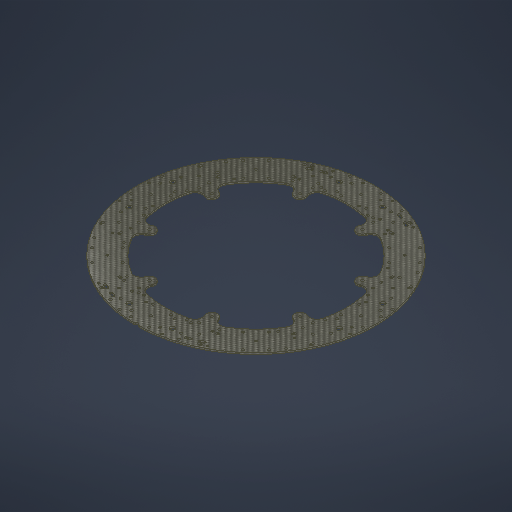
# Autodesk Inventor part: Body_Outer_Plate
Saved by Autodesk Inventor 2025 (Build 290162010, 162A)
## iProperties
Created: 2023-12-04
Part Number: Body_Outer_Plate
Material: CFRP
Document SubType Name: Modeling
Designer: dzw04
Density: 1.43 g/cm^3
Appearance: Carbon Fiber 1
Mass: 106.561 g
Surface Area: 824.877 cm^2
Volume: 74.5179 cm^3
Author: dzw04
Autodesk Inventor part; units mm, degrees
ref_plane "YZ Plane" through (0, 0, 0) normal (1, 0, 0) x (0, 1, 0)
ref_plane "XZ Plane" through (0, 0, 0) normal (0, 1, 0) x (-1, 0, 0)
ref_plane "XY Plane" through (0, 0, 0) normal (0, 0, 1) x (1, 0, 0)
sketch "Sketch1" plane through (0, 0, 0) normal (0, 1, 0) x (-1, 0, 0)
  arc A0 (286.4193, 194.7045) -> (272.8789, 201.567) centre (276.7057, 192.3282) ccw
  arc A1 (201.1228, 271.8066) -> (214.981, 266.0663) centre (208.0519, 268.9364) ccw
  line L0 (215.4252, 267.1386) -> (214.981, 266.0663)
  arc A2 (229.8521, 271.8607) -> (215.4252, 267.1386) centre (224.664, 263.3118) ccw
  circle A3 centre (39.4263, 92.5) radius 1.6
  circle A4 centre (61.0636, 208.0519) radius 1.6
  circle A5 centre (165, 310) radius 1.6
  arc A6 (271.8607, 229.8521) -> (229.8521, 271.8607) centre (165, 165) ccw
  circle A7 centre (267.5305, 62.4695) radius 1.6
  arc A8 (58.1393, 229.8521) -> (62.8614, 215.4252) centre (66.6882, 224.664) ccw
  arc A9 (267.1386, 215.4252) -> (271.8607, 229.8521) centre (263.3118, 224.664) ccw
  line L1 (266.0663, 214.981) -> (267.1386, 215.4252)
  circle A10 centre (290.5737, 92.5) radius 1.6
  arc A11 (266.0663, 214.981) -> (271.8066, 201.1228) centre (268.9364, 208.0519) ccw
  line L2 (272.8789, 201.567) -> (271.8066, 201.1228)
  circle A12 centre (109.5109, 298.9625) radius 1.6
  line L3 (201.567, 57.1211) -> (201.1228, 58.1934)
  circle A13 centre (121.9481, 268.9364) radius 1.6
  arc A14 (286.4193, 135.2955) -> (286.4193, 194.7045) centre (165, 165) ccw
  arc A15 (272.8789, 128.433) -> (286.4193, 135.2955) centre (276.7057, 137.6718) ccw
  circle A16 centre (31.0375, 109.5109) radius 1.6
  line L4 (271.8066, 128.8772) -> (272.8789, 128.433)
  arc A17 (271.8066, 128.8772) -> (266.0663, 115.019) centre (268.9364, 121.9481) ccw
  circle A18 centre (109.5109, 31.0375) radius 1.6
  circle A19 centre (62.4695, 267.5305) radius 1.6
  line L5 (267.1386, 114.5748) -> (266.0663, 115.019)
  arc A20 (271.8607, 100.1479) -> (267.1386, 114.5748) centre (263.3118, 105.336) ccw
  arc A21 (229.8521, 58.1393) -> (271.8607, 100.1479) centre (165, 165) ccw
  circle A22 centre (268.9364, 208.0519) radius 1.6
  arc A23 (215.4252, 62.8614) -> (229.8521, 58.1393) centre (224.664, 66.6882) ccw
  line L6 (214.981, 63.9337) -> (215.4252, 62.8614)
  arc A24 (214.981, 63.9337) -> (201.1228, 58.1934) centre (208.0519, 61.0636) ccw
  line L7 (62.8614, 215.4252) -> (63.9337, 214.981)
  arc A25 (194.7045, 43.5807) -> (201.567, 57.1211) centre (192.3282, 53.2943) ccw
  arc A26 (135.2955, 43.5807) -> (194.7045, 43.5807) centre (165, 165) ccw
  arc A27 (128.433, 57.1211) -> (135.2955, 43.5807) centre (137.6718, 53.2943) ccw
  line L8 (128.8772, 58.1934) -> (128.433, 57.1211)
  circle A28 centre (39.4263, 237.5) radius 1.6
  circle A29 centre (31.0375, 220.4891) radius 1.6
  arc A30 (58.1934, 201.1228) -> (63.9337, 214.981) centre (61.0636, 208.0519) ccw
  arc A31 (128.8772, 58.1934) -> (115.019, 63.9337) centre (121.9481, 61.0636) ccw
  circle A32 centre (62.4695, 62.4695) radius 1.6
  line L9 (114.5748, 62.8614) -> (115.019, 63.9337)
  circle A33 centre (20, 165) radius 1.6
  arc A34 (100.1479, 58.1393) -> (114.5748, 62.8614) centre (105.336, 66.6882) ccw
  circle A35 centre (267.5305, 267.5305) radius 1.6
  line L10 (58.1934, 201.1228) -> (57.1211, 201.567)
  arc A36 (57.1211, 201.567) -> (43.5807, 194.7045) centre (53.2943, 192.3282) ccw
  circle A37 centre (61.0636, 121.9481) radius 1.6
  circle A38 centre (298.9625, 220.4891) radius 1.6
  arc A39 (43.5807, 194.7045) -> (43.5807, 135.2955) centre (165, 165) ccw
  arc A40 (43.5807, 135.2955) -> (57.1211, 128.433) centre (53.2943, 137.6718) ccw
  line L11 (57.1211, 128.433) -> (58.1934, 128.8772)
  arc A41 (63.9337, 115.019) -> (58.1934, 128.8772) centre (61.0636, 121.9481) ccw
  circle A42 centre (208.0519, 61.0636) radius 1.6
  circle A43 centre (298.9625, 109.5109) radius 1.6
  circle A44 centre (220.4891, 31.0375) radius 1.6
  line L12 (63.9337, 115.019) -> (62.8614, 114.5748)
  circle A45 centre (165, 20) radius 1.6
  arc A46 (62.8614, 114.5748) -> (58.1393, 100.1479) centre (66.6882, 105.336) ccw
  circle A47 centre (208.0519, 268.9364) radius 1.6
  arc A48 (58.1393, 100.1479) -> (100.1479, 58.1393) centre (165, 165) ccw
  circle A49 centre (268.9364, 121.9481) radius 1.6
  circle A50 centre (310, 165) radius 1.6
  arc A51 (162.8516, 328.7216) -> (167.1484, 328.7216) centre (165, 330) ccw
  arc A52 (162.8516, 328.7216) -> (160.6371, 329.9423) centre (160.7032, 327.4432) ccw
  arc A53 (169.3629, 329.9423) -> (167.1484, 328.7216) centre (169.2968, 327.4432) ccw
  line L13 (115.019, 266.0663) -> (114.5748, 267.1386)
  circle A54 centre (290.5737, 237.5) radius 1.6
  circle A55 centre (220.4891, 298.9625) radius 1.6
  circle A56 centre (121.9481, 61.0636) radius 1.6
  arc A57 (160.6371, 329.9423) -> (169.3629, 329.9423) centre (165, 165) ccw
  circle A58 centre (135.5551, 323.917) radius 1.6
  circle A59 centre (135.5551, 289.917) radius 1.6
  circle A60 centre (194.4449, 289.917) radius 1.6
  circle A61 centre (194.4449, 323.917) radius 1.6
  circle A62 centre (6.083, 135.5551) radius 1.6
  circle A63 centre (40.083, 135.5551) radius 1.6
  circle A64 centre (40.083, 194.4449) radius 1.6
  circle A65 centre (6.083, 194.4449) radius 1.6
  circle A66 centre (194.4449, 6.083) radius 1.6
  circle A67 centre (194.4449, 40.083) radius 1.6
  circle A68 centre (135.5551, 40.083) radius 1.6
  circle A69 centre (135.5551, 6.083) radius 1.6
  circle A70 centre (323.917, 194.4449) radius 1.6
  circle A71 centre (289.917, 194.4449) radius 1.6
  circle A72 centre (289.917, 135.5551) radius 1.6
  circle A73 centre (323.917, 135.5551) radius 1.6
  arc A74 (201.567, 272.8789) -> (194.7045, 286.4193) centre (192.3282, 276.7057) ccw
  line L14 (201.1228, 271.8066) -> (201.567, 272.8789)
  arc A75 (194.7045, 286.4193) -> (135.2955, 286.4193) centre (165, 165) ccw
  arc A76 (135.2955, 286.4193) -> (128.433, 272.8789) centre (137.6718, 276.7057) ccw
  line L15 (128.433, 272.8789) -> (128.8772, 271.8066)
  arc A77 (115.019, 266.0663) -> (128.8772, 271.8066) centre (121.9481, 268.9364) ccw
  arc A78 (114.5748, 267.1386) -> (100.1479, 271.8607) centre (105.336, 263.3118) ccw
  arc A79 (100.1479, 271.8607) -> (58.1393, 229.8521) centre (165, 165) ccw
  circle A80 centre (212.3712, 318.561) radius 1.6
  circle A81 centre (200.8907, 39.1554) radius 1.6
  circle A82 centre (117.6288, 318.561) radius 1.6
  circle A83 centre (89.9125, 307.0805) radius 1.6
  circle A84 centre (101.393, 279.3641) radius 1.6
  circle A85 centre (200.8907, 290.8446) radius 1.6
  circle A86 centre (104.0989, 285.8969) radius 1.6
  circle A87 centre (129.1093, 290.8446) radius 1.6
  circle A88 centre (240.0875, 307.0805) radius 1.6
  circle A89 centre (228.607, 279.3641) radius 1.6
  circle A90 centre (225.9011, 285.8969) radius 1.6
  circle A91 centre (207.4235, 293.5506) radius 1.6
  circle A92 centre (117.6288, 11.439) radius 1.6
  circle A93 centre (89.9125, 22.9195) radius 1.6
  circle A94 centre (101.393, 50.6359) radius 1.6
  circle A95 centre (104.0989, 44.1031) radius 1.6
  circle A96 centre (122.5765, 36.4494) radius 1.6
  circle A97 centre (129.1093, 39.1554) radius 1.6
  circle A98 centre (212.3712, 11.439) radius 1.6
  circle A99 centre (240.0875, 22.9195) radius 1.6
  circle A100 centre (228.607, 50.6359) radius 1.6
  circle A101 centre (225.9011, 44.1031) radius 1.6
  circle A102 centre (207.4235, 36.4494) radius 1.6
  line L16 (17.2755, 136.1225) -> (17.2755, 133.8775)
  line L17 (17.2755, 196.1225) -> (17.2755, 193.8775)
  arc A103 (18.3955, 192.0815) -> (18.3955, 197.9185) centre (19.8255, 195) ccw
  arc A104 (132.0815, 311.6045) -> (137.9185, 311.6045) centre (135, 310.1745) ccw
  arc A105 (192.0815, 311.6045) -> (197.9185, 311.6045) centre (195, 310.1745) ccw
  line L18 (196.1225, 312.7245) -> (193.8775, 312.7245)
  arc A106 (311.6045, 197.9185) -> (311.6045, 192.0815) centre (310.1745, 195) ccw
  line L19 (312.7245, 193.8775) -> (312.7245, 196.1225)
  arc A107 (311.6045, 137.9185) -> (311.6045, 132.0815) centre (310.1745, 135) ccw
  line L20 (312.7245, 133.8775) -> (312.7245, 136.1225)
  arc A108 (197.9185, 18.3955) -> (192.0815, 18.3955) centre (195, 19.8255) ccw
  line L21 (193.8775, 17.2755) -> (196.1225, 17.2755)
  line L22 (133.8775, 17.2755) -> (136.1225, 17.2755)
  arc A109 (137.9185, 18.3955) -> (132.0815, 18.3955) centre (135, 19.8255) ccw
  line L23 (136.1225, 312.7245) -> (133.8775, 312.7245)
  arc A110 (18.3955, 132.0815) -> (18.3955, 137.9185) centre (19.8255, 135) ccw
  circle A111 centre (32.6859, 255.8253) radius 1.6
  circle A112 centre (152.5, 295) radius 1.6
  circle A113 centre (64.2373, 81.915) radius 1.6
  circle A114 centre (60.7017, 286.9759) radius 1.6
  circle A115 centre (43.0241, 269.2983) radius 1.6
  circle A116 centre (58.6667, 89.1747) radius 1.6
  circle A117 centre (297.3141, 74.1747) radius 1.6
  circle A118 centre (81.915, 64.2373) radius 1.6
  circle A119 centre (269.2983, 286.9759) radius 1.6
  circle A120 centre (43.0241, 60.7017) radius 1.6
  circle A121 centre (152.5, 35) radius 1.6
  circle A122 centre (81.915, 265.7627) radius 1.6
  circle A123 centre (295, 152.5) radius 1.6
  circle A124 centre (177.5, 35) radius 1.6
  circle A125 centre (283.8333, 219.1747) radius 1.6
  circle A126 centre (64.2373, 248.085) radius 1.6
  circle A127 centre (271.3333, 240.8253) radius 1.6
  circle A128 centre (297.3141, 255.8253) radius 1.6
  circle A129 centre (5, 152.5) radius 1.6
  circle A130 centre (283.8333, 110.8253) radius 1.6
  circle A131 centre (295, 177.5) radius 1.6
  circle A132 centre (177.5, 5) radius 1.6
  circle A133 centre (271.3333, 89.1747) radius 1.6
  circle A134 centre (286.9759, 269.2983) radius 1.6
  circle A135 centre (177.5, 295) radius 1.6
  circle A136 centre (60.7017, 43.0241) radius 1.6
  circle A137 centre (325, 152.5) radius 1.6
  circle A138 centre (152.5, 325) radius 1.6
  circle A139 centre (325, 177.5) radius 1.6
  circle A140 centre (32.6859, 74.1747) radius 1.6
  circle A141 centre (35, 152.5) radius 1.6
  circle A142 centre (286.9759, 60.7017) radius 1.6
  circle A143 centre (265.7627, 81.915) radius 1.6
  circle A144 centre (46.1667, 110.8253) radius 1.6
  circle A145 centre (269.2983, 43.0241) radius 1.6
  circle A146 centre (265.7627, 248.085) radius 1.6
  circle A147 centre (152.5, 5) radius 1.6
  circle A148 centre (248.085, 64.2373) radius 1.6
  circle A149 centre (177.5, 325) radius 1.6
  circle A150 centre (46.1667, 219.1747) radius 1.6
  circle A151 centre (35, 177.5) radius 1.6
  circle A152 centre (5, 177.5) radius 1.6
  circle A153 centre (58.6667, 240.8253) radius 1.6
  circle A154 centre (248.085, 265.7627) radius 1.6
  arc A155 (308.4, 231.6) -> (311.6, 231.6) centre (310, 231.6) ccw
  arc A156 (311.6, 233.4) -> (311.4139, 234.149) centre (310, 233.4) ccw
  line L24 (311.6, 233.4) -> (311.6, 231.6)
  arc A157 (18.5861, 95.851) -> (21.5998, 96.5743) centre (20.1859, 95.8253) ccw
  line L25 (308.4, 231.6) -> (308.4, 233.4)
  arc A158 (308.4002, 233.4257) -> (308.4, 233.4) centre (310, 233.4) ccw
  arc A159 (311.4139, 234.149) -> (308.4002, 233.4257) centre (309.8141, 234.1747) ccw
  arc A160 (311.4139, 95.851) -> (311.6, 96.6) centre (310, 96.6) ccw
  line L26 (311.6, 96.6) -> (311.6, 98.4)
  arc A161 (311.6, 98.4) -> (308.4, 98.4) centre (310, 98.4) ccw
  line L27 (308.4, 98.4) -> (308.4, 96.6)
  arc A162 (308.4, 96.6) -> (308.4002, 96.5743) centre (310, 96.6) ccw
  arc A163 (308.4002, 96.5743) -> (311.4139, 95.851) centre (309.8141, 95.8253) ccw
  arc A164 (18.5861, 234.149) -> (18.4, 233.4) centre (20, 233.4) ccw
  line L28 (18.4, 233.4) -> (18.4, 231.6)
  arc A165 (18.4, 231.6) -> (21.6, 231.6) centre (20, 231.6) ccw
  line L29 (21.6, 231.6) -> (21.6, 233.4)
  arc A166 (21.6, 233.4) -> (21.5998, 233.4257) centre (20, 233.4) ccw
  arc A167 (21.5998, 233.4257) -> (18.5861, 234.149) centre (20.1859, 234.1747) ccw
  arc A168 (18.4, 96.6) -> (18.5861, 95.851) centre (20, 96.6) ccw
  line L30 (18.4, 96.6) -> (18.4, 98.4)
  arc A169 (21.6, 98.4) -> (18.4, 98.4) centre (20, 98.4) ccw
  line L31 (21.6, 98.4) -> (21.6, 96.6)
  arc A170 (21.5998, 96.5743) -> (21.6, 96.6) centre (20, 96.6) ccw
  arc A171 (231.6, 311.6) -> (231.6, 308.4) centre (231.6, 310) ccw
  arc A172 (98.4, 308.4) -> (98.4, 311.6) centre (98.4, 310) ccw
  line L32 (98.4, 311.6) -> (96.6, 311.6)
  arc A173 (96.6, 21.6) -> (96.6, 18.4) centre (96.6, 20) ccw
  circle A174 centre (123.4, 20) radius 1.6
  arc A175 (96.6, 286.6) -> (96.6, 283.4) centre (96.6, 285) ccw
  line L33 (96.6, 283.4) -> (98.4, 283.4)
  arc A176 (98.4, 283.4) -> (98.4, 286.6) centre (98.4, 285) ccw
  line L34 (98.4, 286.6) -> (96.6, 286.6)
  circle A177 centre (310, 206.6) radius 1.6
  circle A178 centre (285, 206.6) radius 1.6
  arc A179 (283.4, 231.6) -> (286.6, 231.6) centre (285, 231.6) ccw
  line L35 (286.6, 231.6) -> (286.6, 233.4)
  arc A180 (286.6, 233.4) -> (283.4, 233.4) centre (285, 233.4) ccw
  arc A181 (233.4, 43.4) -> (233.4, 46.6) centre (233.4, 45) ccw
  line L36 (283.4, 233.4) -> (283.4, 231.6)
  circle A182 centre (206.6, 45) radius 1.6
  circle A183 centre (206.6, 20) radius 1.6
  arc A184 (233.4, 18.4) -> (233.4, 21.6) centre (233.4, 20) ccw
  line L37 (233.4, 21.6) -> (231.6, 21.6)
  arc A185 (231.6, 21.6) -> (231.6, 18.4) centre (231.6, 20) ccw
  circle A186 centre (123.4, 45) radius 1.6
  line L38 (231.6, 43.4) -> (233.4, 43.4)
  arc A187 (231.6, 46.6) -> (231.6, 43.4) centre (231.6, 45) ccw
  circle A188 centre (206.6, 285) radius 1.6
  circle A189 centre (206.6, 310) radius 1.6
  arc A190 (233.4, 308.4) -> (233.4, 311.6) centre (233.4, 310) ccw
  line L39 (233.4, 308.4) -> (231.6, 308.4)
  line L40 (231.6, 18.4) -> (233.4, 18.4)
  line L41 (231.6, 311.6) -> (233.4, 311.6)
  arc A191 (233.4, 283.4) -> (233.4, 286.6) centre (233.4, 285) ccw
  line L42 (233.4, 283.4) -> (231.6, 283.4)
  arc A192 (231.6, 286.6) -> (231.6, 283.4) centre (231.6, 285) ccw
  line L43 (233.4, 46.6) -> (231.6, 46.6)
  circle A193 centre (123.4, 285) radius 1.6
  circle A194 centre (123.4, 310) radius 1.6
  arc A195 (96.6, 311.6) -> (96.6, 308.4) centre (96.6, 310) ccw
  line L44 (96.6, 308.4) -> (98.4, 308.4)
  line L45 (96.6, 21.6) -> (98.4, 21.6)
  arc A196 (98.4, 18.4) -> (98.4, 21.6) centre (98.4, 20) ccw
  line L46 (98.4, 18.4) -> (96.6, 18.4)
  arc A197 (96.6, 46.6) -> (96.6, 43.4) centre (96.6, 45) ccw
  line L47 (96.6, 46.6) -> (98.4, 46.6)
  arc A198 (98.4, 43.4) -> (98.4, 46.6) centre (98.4, 45) ccw
  line L48 (98.4, 43.4) -> (96.6, 43.4)
  circle A199 centre (310, 123.4) radius 1.6
  circle A200 centre (285, 123.4) radius 1.6
  arc A201 (286.6, 98.4) -> (283.4, 98.4) centre (285, 98.4) ccw
  line L49 (286.6, 98.4) -> (286.6, 96.6)
  arc A202 (283.4, 96.6) -> (286.6, 96.6) centre (285, 96.6) ccw
  line L50 (283.4, 96.6) -> (283.4, 98.4)
  line L51 (231.6, 286.6) -> (233.4, 286.6)
  circle A203 centre (20, 206.6) radius 1.6
  circle A204 centre (45, 206.6) radius 1.6
  arc A205 (43.4, 231.6) -> (46.6, 231.6) centre (45, 231.6) ccw
  line L52 (43.4, 231.6) -> (43.4, 233.4)
  arc A206 (46.6, 233.4) -> (43.4, 233.4) centre (45, 233.4) ccw
  line L53 (46.6, 233.4) -> (46.6, 231.6)
  circle A207 centre (20, 123.4) radius 1.6
  circle A208 centre (45, 123.4) radius 1.6
  arc A209 (46.6, 98.4) -> (43.4, 98.4) centre (45, 98.4) ccw
  line L54 (43.4, 98.4) -> (43.4, 96.6)
  arc A210 (43.4, 96.6) -> (46.6, 96.6) centre (45, 96.6) ccw
  line L55 (46.6, 96.6) -> (46.6, 98.4)
  arc A211 (97.0576, 27.1037) -> (95.833, 24.1473) centre (96.4453, 25.6255) ccw
  line L56 (97.0576, 27.1037) -> (101.677, 25.1903)
  arc A212 (100.4524, 22.2339) -> (101.677, 25.1903) centre (101.0647, 23.7121) ccw
  arc A213 (214.4648, 19.45) -> (215.6894, 16.4936) centre (215.0771, 17.9718) ccw
  arc A214 (220.3088, 18.407) -> (219.0842, 21.3635) centre (219.6965, 19.8853) ccw
  line L57 (220.3088, 18.407) -> (215.6894, 16.4936)
  arc A215 (228.323, 25.1903) -> (229.5476, 22.2339) centre (228.9353, 23.7121) ccw
  arc A216 (115.5352, 310.55) -> (114.3106, 313.5064) centre (114.9229, 312.0282) ccw
  line L58 (110.9158, 308.6365) -> (115.5352, 310.55)
  arc A217 (109.6912, 311.593) -> (110.9158, 308.6365) centre (110.3035, 310.1147) ccw
  line L59 (228.323, 25.1903) -> (232.9424, 27.1037)
  arc A218 (234.167, 24.1473) -> (232.9424, 27.1037) centre (233.5547, 25.6255) ccw
  line L60 (234.167, 24.1473) -> (229.5476, 22.2339)
  line L61 (214.4648, 19.45) -> (219.0842, 21.3635)
  arc A219 (232.9424, 302.8963) -> (234.167, 305.8527) centre (233.5547, 304.3745) ccw
  line L62 (228.323, 304.8097) -> (232.9424, 302.8963)
  line L63 (114.3106, 313.5064) -> (109.6912, 311.593)
  arc A220 (101.677, 304.8097) -> (100.4524, 307.7661) centre (101.0647, 306.2879) ccw
  line L64 (97.0576, 302.8963) -> (101.677, 304.8097)
  arc A221 (95.833, 305.8527) -> (97.0576, 302.8963) centre (96.4453, 304.3745) ccw
  line L65 (100.4524, 307.7661) -> (95.833, 305.8527)
  arc A222 (229.5476, 307.7661) -> (228.323, 304.8097) centre (228.9353, 306.2879) ccw
  line L66 (114.3106, 16.4936) -> (109.6912, 18.407)
  arc A223 (110.9158, 21.3635) -> (109.6912, 18.407) centre (110.3035, 19.8853) ccw
  line L67 (110.9158, 21.3635) -> (115.5352, 19.45)
  arc A224 (114.3106, 16.4936) -> (115.5352, 19.45) centre (114.9229, 17.9718) ccw
  line L68 (100.4524, 22.2339) -> (95.833, 24.1473)
  line L69 (220.3088, 311.593) -> (215.6894, 313.5064)
  arc A225 (219.0842, 308.6365) -> (220.3088, 311.593) centre (219.6965, 310.1147) ccw
  line L70 (214.4648, 310.55) -> (219.0842, 308.6365)
  arc A226 (215.6894, 313.5064) -> (214.4648, 310.55) centre (215.0771, 312.0282) ccw
  line L71 (234.167, 305.8527) -> (229.5476, 307.7661)
  circle A227 centre (185, 296.917) radius 1.6
  circle A228 centre (185, 33.083) radius 1.6
  circle A229 centre (33.083, 185) radius 1.6
  circle A230 centre (145, 316.917) radius 1.6
  circle A231 centre (185, 13.083) radius 1.6
  circle A232 centre (13.083, 185) radius 1.6
  circle A233 centre (33.083, 145) radius 1.6
  circle A234 centre (13.083, 145) radius 1.6
  circle A235 centre (185, 316.917) radius 1.6
  circle A236 centre (145, 13.083) radius 1.6
  circle A237 centre (316.917, 185) radius 1.6
  circle A238 centre (296.917, 185) radius 1.6
  circle A239 centre (296.917, 145) radius 1.6
  circle A240 centre (316.917, 145) radius 1.6
  circle A241 centre (145, 33.083) radius 1.6
  circle A242 centre (145, 296.917) radius 1.6
  arc A243 (311.6045, 132.0815) -> (312.7245, 133.8775) centre (310.7245, 133.8775) ccw
  arc A244 (312.7245, 136.1225) -> (311.6045, 137.9185) centre (310.7245, 136.1225) ccw
  arc A245 (312.7245, 196.1225) -> (311.6045, 197.9185) centre (310.7245, 196.1225) ccw
  arc A246 (311.6045, 192.0815) -> (312.7245, 193.8775) centre (310.7245, 193.8775) ccw
  arc A247 (197.9185, 311.6045) -> (196.1225, 312.7245) centre (196.1225, 310.7245) ccw
  arc A248 (193.8775, 312.7245) -> (192.0815, 311.6045) centre (193.8775, 310.7245) ccw
  arc A249 (137.9185, 311.6045) -> (136.1225, 312.7245) centre (136.1225, 310.7245) ccw
  arc A250 (133.8775, 312.7245) -> (132.0815, 311.6045) centre (133.8775, 310.7245) ccw
  arc A251 (18.3955, 197.9185) -> (17.2755, 196.1225) centre (19.2755, 196.1225) ccw
  arc A252 (17.2755, 193.8775) -> (18.3955, 192.0815) centre (19.2755, 193.8775) ccw
  arc A253 (17.2755, 133.8775) -> (18.3955, 132.0815) centre (19.2755, 133.8775) ccw
  arc A254 (18.3955, 137.9185) -> (17.2755, 136.1225) centre (19.2755, 136.1225) ccw
  arc A255 (132.0815, 18.3955) -> (133.8775, 17.2755) centre (133.8775, 19.2755) ccw
  arc A256 (136.1225, 17.2755) -> (137.9185, 18.3955) centre (136.1225, 19.2755) ccw
  arc A257 (192.0815, 18.3955) -> (193.8775, 17.2755) centre (193.8775, 19.2755) ccw
  arc A258 (196.1225, 17.2755) -> (197.9185, 18.3955) centre (196.1225, 19.2755) ccw
  point P0 (17.2755, 137.0149)
  point P1 (17.2755, 132.9851)
  point P2 (17.2755, 197.0149)
  point P3 (17.2755, 192.9851)
  point P4 (17.2755, 192.9851)
  point P5 (17.2755, 197.0149)
  point P6 (132.9851, 312.7245)
  point P7 (137.0149, 312.7245)
  point P8 (192.9851, 312.7245)
  point P9 (197.0149, 312.7245)
  point P10 (197.0149, 312.7245)
  point P11 (192.9851, 312.7245)
  point P12 (312.7245, 197.0149)
  point P13 (312.7245, 192.9851)
  point P14 (312.7245, 192.9851)
  point P15 (312.7245, 197.0149)
  point P16 (312.7245, 137.0149)
  point P17 (312.7245, 132.9851)
  point P18 (312.7245, 132.9851)
  point P19 (312.7245, 137.0149)
  point P20 (197.0149, 17.2755)
  point P21 (192.9851, 17.2755)
  point P22 (192.9851, 17.2755)
  point P23 (197.0149, 17.2755)
  point P24 (132.9851, 17.2755)
  point P25 (137.0149, 17.2755)
  point P26 (137.0149, 17.2755)
  point P27 (132.9851, 17.2755)
  point P28 (137.0149, 312.7245)
  point P29 (132.9851, 312.7245)
  point P30 (17.2755, 132.9851)
  point P31 (17.2755, 137.0149)
  point P32 (167.1484, 328.7216)
  point P33 (100.4524, 307.7661)
  point P34 (232.9424, 302.8963)
  point P35 (234.167, 305.8527)
  point P36 (109.6912, 311.593)
  point P37 (114.3106, 313.5064)
  point P38 (234.167, 24.1473)
  point P39 (229.5476, 22.2339)
  point P40 (215.6894, 16.4936)
  point P41 (214.4648, 19.45)
  point P42 (219.0842, 21.3635)
  point P43 (95.833, 24.1473)
  point P44 (97.0576, 27.1037)
  point P45 (46.6, 98.4)
  point P46 (46.6, 96.6)
  point P47 (46.6, 233.4)
  point P48 (46.6, 231.6)
  point P49 (18.5861, 234.149)
  point P50 (308.4002, 96.5743)
  point P51 (21.5998, 96.5743)
  point P52 (137.0149, 17.2755)
  point P53 (132.9851, 17.2755)
  point P54 (192.9851, 17.2755)
  point P55 (197.0149, 17.2755)
  point P56 (312.7245, 132.9851)
  point P57 (312.7245, 137.0149)
  point P58 (312.7245, 192.9851)
  point P59 (312.7245, 197.0149)
  point P60 (197.0149, 312.7245)
  point P61 (192.9851, 312.7245)
  point P62 (137.0149, 312.7245)
  point P63 (132.9851, 312.7245)
  point P64 (17.2755, 192.9851)
  point P65 (17.2755, 197.0149)
  point P66 (17.2755, 132.9851)
  point P67 (17.2755, 137.0149)
  point P68 (271.8066, 128.8772)
  point P69 (266.0663, 115.019)
  point P70 (271.8607, 100.1479)
  point P71 (229.8521, 58.1393)
  point P72 (215.4252, 62.8614)
  point P73 (194.7045, 43.5807)
  point P74 (135.2955, 43.5807)
  point P75 (115.019, 63.9337)
  point P76 (58.1393, 100.1479)
  point P77 (63.9337, 115.019)
  point P78 (57.1211, 128.433)
  point P79 (43.5807, 135.2955)
  point P80 (62.8614, 215.4252)
  point P81 (58.1393, 229.8521)
  point P82 (100.1479, 271.8607)
  point P83 (135.2955, 286.4193)
  point P84 (201.1228, 271.8066)
  point P85 (214.981, 266.0663)
  point P86 (267.1386, 215.4252)
  point P87 (266.0663, 214.981)
  point P88 (271.8066, 201.1228)
  point P89 (286.4193, 194.7045)
  dimension "d2" = 2
  constraints: 259 centre point, 248 point on circle, 144 end point, 32 tangent, 16 point on line, 15 equal radius
  measures "d2" radius of A243
extrude "Extrusion1" add sketch "Sketch1" along normal blind 2
equation "\"d0\" = ThicknessBodyOuterPlate"
equation "\"MountToMotorCenter\" = 0"
equation "\"ArmPosition\" = 5deg"
equation "\"BatteryWidth\" = 62"
equation "\"BatteryHeight\" = 76"
equation "\"ThicknessBodyOuterPlate\" = 2"
equation "\"ThicknessBodyCenterPlate\" = 2"
equation "\"ThicknessLegLoadpipePlate\" = 2"
equation "\"ThicknessBatteryTray\" = 2"
equation "\"ThicknessBatteryTopTray\" = 1"
equation "\"LandingGearStabilityBar\" = 525"
equation "\"StartAngleArm\" = 45deg"
equation "\"MotorMountCenter\" = 71.5"
body "Solid1"
